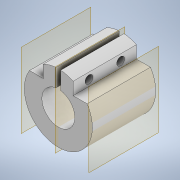
# Autodesk Inventor part: Cuff
Saved by Autodesk Inventor 2021 (Build 250183000, 183)
## iProperties
Created: 2021-04-08
Part Number: Cuff
Material: Generic
Document SubType Name: Modeling
Designer: Olivi
Density: 1 g/cm^3
Appearance: Default
Author: Olivi
Autodesk Inventor part; units mm, degrees
ref_plane "YZ Plane" through (0, 0, 0) normal (1, 0, 0) x (0, 1, 0)
ref_plane "XZ Plane" through (0, 0, 0) normal (0, 1, 0) x (-1, 0, 0)
ref_plane "XY Plane" through (0, 0, 0) normal (0, 0, 1) x (1, 0, 0)
sketch "Sketch1" plane through (0, 0, 0) normal (0, 0, 1) x (1, 0, 0)
  point P0 (0, 0)
sketch "Sketch2" plane through (0, 0, 0) normal (0, 0, 1) x (1, 0, 0)
  circle A0 centre (0, 0) radius 10.4
  circle A1 centre (0, 0) radius 21.5
  line L0 (0, 10.0548) -> (-1.5, 10.0548)
  line L1 (-1.5, 10.0548) -> (-1.5, 22.3246)
  line L2 (-1.5, 22.3246) -> (1.5, 22.3246)
  line L3 (1.5, 22.3246) -> (1.5, 10.0548)
  line L4 (1.5, 10.0548) -> (0, 10.0548)
  point P0 (1.5, 21.4476)
  point P1 (1.5, 10.2913)
  point P2 (-1.5, 10.2913)
  point P3 (-1.5, 21.4476)
  dimension "d0" = 20.8
  dimension "d1" = 43
  dimension "d3" = 1.5
  dimension "d4" = 3
  constraints: 10 end point, 4 perpendicular, 2 centre point, 2 coincident, 1 horizontal, 1 point on line
  measures "d0" diameter of A0
  measures "d1" diameter of A1
  measures "d3" distance of L0.start L0.end
  measures "d4" distance of L1.end L2.end
extrude "Extrusion1" add sketch "Sketch2" along normal blind 40 contours A0 L3 A1 L1 picked at (17.4874, -2.5592)
ref_plane "Work Plane1" through (0, 10.2913, 0) normal (1, 0, 0) x (0, 0, -1)
ref_plane "Work Plane2" through (21.35, 10.2913, 0) normal (1, 0, 0) x (0, 0, -1)
sketch "Sketch3" plane through (21.35, 10.2913, 0) normal (1, 0, 0) x (0, 0, -1)
  line L0 (-40, 0) -> (-40, 11.1564) projected
  line L1 (-40, 11.1564) -> (-40, 1.1564)
  line L2 (-40, 1.1564) -> (0, 1.1564)
  line L3 (0, 0) -> (-40, 0) projected
  line L4 (0, 0) -> (0, 11.1564) projected
  line L5 (0, 1.1564) -> (0, 11.1564)
  line L6 (0, 11.1564) -> (-40, 11.1564) projected
  line L7 (0, 11.1564) -> (-40, 11.1564)
  point P0 (0, -10.2913)
  dimension "d8" = 10
  constraints: 8 end point, 1 collinear, 1 parallel, 1 perpendicular, 1 point on line
  measures "d8" distance of L0.end L1.end
extrude "Extrusion2" cut sketch "Sketch3" against normal blind 12 contours L0 L6 L4 L2
ref_plane "Work Plane3" through (-21.5, 10.2913, 0) normal (1, 0, 0) x (0, 0, -1)
sketch "Sketch4" plane through (-21.5, 10.2913, 0) normal (1, 0, 0) x (0, 0, -1)
  line L0 (0, 11.1564) -> (-40, 11.1564) projected
  line L1 (0, 11.1564) -> (0, 1.1564)
  line L2 (0, 11.1564) -> (0, 0) projected
  line L3 (0, 1.1564) -> (-40, 1.1564)
  line L4 (-40, 0) -> (-40, 11.1564) projected
  line L5 (-40, 11.1564) -> (0, 11.1564)
  point P0 (0, -10.2913)
  dimension "d12" = 10
  constraints: 6 end point, 2 point on line, 1 parallel, 1 perpendicular
  measures "d12" distance of L0.start L1.end
extrude "Extrusion3" cut sketch "Sketch4" along normal blind 12
sketch "Sketch5" plane through (9.35, 10.2913, 0) normal (1, 0, 0) x (0, 0, -1)
  circle A0 centre (-30, 5.0692) radius 2.5
  circle A1 centre (-10, 5.0692) radius 2.5
  line L0 (-40, 1.1564) -> (-40, 9.0692) projected
  line L1 (0, 9.0692) -> (0, 1.1564) projected
  line L2 (-40, 9.0692) -> (0, 9.0692) projected
  point P0 (0, -10.2913)
  dimension "d15" = 5
  dimension "d16" = 5
  dimension "d17" = 10
  dimension "d18" = 10
  dimension "d19" = 4
  dimension "d20" = 4
  constraints: 2 centre point
  measures "d15" diameter of A0
  measures "d16" diameter of A1
  measures "d17" distance from line of L0 A0.centre
  measures "d18" distance from line of L1 A1.centre
  measures "d19" distance from line of L2 A0.centre
  measures "d20" distance from line of L2 A1.centre
extrude "Extrusion4" cut sketch "Sketch5" against normal through all
body "Solid1"
